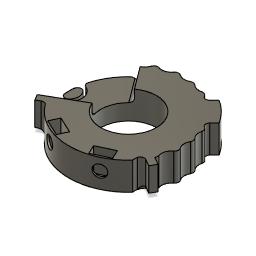
thumbwheelSmall (Autodesk Fusion 360 design; units mm, degrees)
Autodesk Fusion 360 part; units mm, degrees
sketch "Sketch1" plane through (0, 0, 0) normal (0, 1, 0) x (1, 0, 0)
  circle A0 centre (0, 0) radius 7
  circle A1 centre (0, 0) radius 15
  line L0 (0, -32.8401) -> (0, 23.247)
  line L1 (-28.2843, 0) -> (28.2843, 0)
  line L2 (6.3393, 13.5946) -> (-6.3393, -13.5946)
  line L3 (6.3393, 13.5946) -> (-6.3393, -13.5946)
  line L4 (-6.3393, 13.5946) -> (6.3393, -13.5946)
  circle A2 centre (-15, 0) radius 2.5
  circle A3 centre (-15, 0) radius 3.25
  circle A4 centre (0, 16.5) radius 2.5
  circle A5 centre (4.2705, 15.9378) radius 2.5
  circle A6 centre (8.25, 14.2894) radius 2.5
  circle A7 centre (11.6673, 11.6673) radius 2.5
  circle A8 centre (14.2894, 8.25) radius 2.5
  circle A9 centre (15.9378, 4.2705) radius 2.5
  circle A10 centre (16.5, 0) radius 2.5
  circle A11 centre (0, 0) radius 16.5
  circle A12 centre (-4.9423, 15.7424) radius 2.5
  circle A13 centre (15.7424, -4.9423) radius 2.5
  circle A14 centre (-9.4307, 13.5393) radius 2.5
  circle A15 centre (13.5393, -9.4307) radius 2.5
  line L5 (-4.0888, -14.0924) -> (-8.1672, -12.1906)
  line L6 (-8.1672, -12.1906) -> (-7.1106, -9.9248)
  line L7 (-7.1106, -9.9248) -> (-3.0322, -11.8266)
  line L8 (-3.0322, -11.8266) -> (-4.0888, -14.0924)
  line L9 (-4.0888, -14.0924) -> (-7.1106, -9.9248) construction
  line L10 (-8.1672, -12.1906) -> (-3.0322, -11.8266) construction
  line L11 (4.0888, -14.0924) -> (8.1672, -12.1906)
  line L12 (7.1106, -9.9248) -> (3.0322, -11.8266)
  line L13 (4.0888, -14.0924) -> (7.1106, -9.9248) construction
  line L14 (3.0322, -11.8266) -> (4.0888, -14.0924)
  line L15 (8.1672, -12.1906) -> (3.0322, -11.8266) construction
  line L16 (8.1672, -12.1906) -> (7.1106, -9.9248)
  line L17 (0, 0) -> (11.6673, 11.6673)
  line L18 (12.0629, 7.1131) -> (7.1131, 12.0629)
  line L19 (7.1131, 12.0629) -> (11.2717, 16.2214)
  line L20 (11.2717, 16.2214) -> (16.2214, 11.2717)
  line L21 (16.2214, 11.2717) -> (12.0629, 7.1131)
  line L22 (12.0629, 7.1131) -> (11.2717, 16.2214) construction
  line L23 (7.1131, 12.0629) -> (16.2214, 11.2717) construction
  point P0 (-5.5997, -12.0086)
  point P1 (6.3393, -13.5946)
  point P2 (6.3393, -13.5946)
  point P3 (5.5997, -12.0086)
  point P4 (11.6673, 11.6673)
  dimension "d1" = 14
  dimension "d2" = 30
  dimension "d3" = 25
  dimension "d6" = 5
  dimension "d7" = 6.5
  dimension "d8" = 5
  dimension "d10" = -90
  dimension "d36" = 5
  dimension "d37" = 5
  dimension "d38" = 5
  dimension "d39" = 5
  dimension "d47" = 4.5
  dimension "d48" = 2.5
  dimension "d49" = 0.5
  dimension "d60" = 45
  dimension "d61" = 33
  dimension "d62" = 7
  constraint coincident A0.centre A1.centre
  constraint concentric A0 A1
  constraint coincident A0.centre L0
  constraint coincident A0.centre L1
  constraint vertical L0
  constraint horizontal L1
  constraint coincident A0.centre L2
  constraint symmetric L0 L2.start L4.start
  constraint symmetric L0 L2.end P2
  constraint coincident A1 L4.start
  constraint coincident A1 L2.start
  constraint coincident A1 L2.end
  constraint coincident L1 A2.centre
  constraint coincident A1 A2.centre
  constraint concentric A2 A3
  constraint coincident L0 A4.centre
  constraint concentric A0 A11
  constraint coincident A10.centre A11
  constraint coincident A11 A12.centre
  constraint tangent A4 A12
  constraint coincident A11 A13.centre
  constraint coincident A11 A14.centre
  constraint tangent A12 A14
  constraint tangent A10 A13
  constraint coincident A11 A15.centre
  constraint tangent A13 A15
  constraint coincident L3 A0.centre
  constraint perpendicular L5 L6
  constraint parallel L5 L7
  constraint parallel L6 L8
  constraint coincident L9 P0
  constraint coincident L10 P0
  constraint coincident L2 P0
  constraint perpendicular L3 L7
  constraint symmetric L0 L5.start L11.start
  constraint symmetric L0 L5.end L11.end
  constraint symmetric L0 L6.end L12.start
  constraint symmetric L0 L7.end L12.end
  constraint symmetric L0 P0 P3
  constraint coincident P4 A7.centre
  constraint perpendicular L18 L19
  constraint parallel L18 L20
  constraint parallel L19 L21
  constraint coincident A8 L18.start
  constraint coincident L22 P4
  constraint coincident L23 P4
  constraint perpendicular L17 L20
  constraint coincident L3 P0
  measures "d1" diameter of A0
  measures "d2" diameter of A1
  measures "d3" angle of L0 L2
  measures "d6" diameter of A2
  measures "d7" diameter of A3
  measures "d8" diameter of A4
  measures "d36" diameter of A12
  measures "d37" diameter of A13
  measures "d38" diameter of A14
  measures "d39" diameter of A15
  measures "d47" distance of L6.end L7.end
  measures "d48" distance of L5.end L6.end
  measures "d49" distance of L2.end L5
  measures "d60" angle of L1 L17
  measures "d61" diameter of A11
  measures "d62" distance of L19.end L20.end
extrude "Extrude1" add sketch "Sketch1" along normal blind 7 contours A0 A1 L1 L4 A10 A13 A15 L11 L12 L16 | A0 A1 L1 A8 A9 A10 L17 L18 | A0 L2 L3 A6 L17 L18 | A0 A1 L0 L4 L11 L12 L14 | A0 A1 L0 L2 L3 A4 A5 A6 | A1 A6 A7 L17 L18 | A1 A7 A8 L17 L18 | A0 A1 L0 L2 L3 L5 L7 L8 | A0 A1 L0 L4 A4 A12 | A0 A1 L1 L4 A3 A14 | A0 A1 L1 L2 L3 A3 L5 L6 L7 | A1 A7 L17 | A1 A7 L17 | A1 A8 L21 | A1 A6 L19 | A1 A6 A7 A11 L17 | A1 A6 A7 | A1 A7 A8 | A1 A7 A8 A11 L17 | A1 A7 A8 A11 L21 | A1 A6 A7 A11 L19 | A1 L1 A2 | A1 L1 A2 | A6 A7 A11 | A7 A8 A11 picked at (12.3821, 7.9516) picked at (9.9243, 12.8711) picked at (12.8711, 9.9243) makes body 1 at (8.1025, 7, -7.9791) makes body 2 at (-12.801, 2.3333, -1.1893)
sketch "Sketch2" plane through (0, 0, 0) normal (0, -1, 0) x (1, 0, 0)
  arc A0 (8.9269, -13.8766) -> (13.8766, -8.9269) centre (0, 0) ccw
  line L0 (13.8766, -8.9269) -> (12.0629, -7.1131)
  arc A1 (13.8369, -5.7913) -> (12.0629, -7.1131) centre (14.2894, -8.25) ccw
  arc A2 (13.8369, -5.7913) -> (13.8793, -5.6891) centre (0, 0) ccw
  arc A3 (14.8644, -2.0127) -> (13.8793, -5.6891) centre (15.9378, -4.2705) ccw
  arc A4 (14.8644, -2.0127) -> (14.8788, -1.9031) centre (0, 0) ccw
  arc A5 (14.8788, 1.9031) -> (14.8788, -1.9031) centre (16.5, 0) ccw
  arc A6 (14.8788, 1.9031) -> (14.7657, 2.641) centre (0, 0) ccw
  arc A7 (13.6256, 6.2724) -> (14.7657, 2.641) centre (15.7424, 4.9423) ccw
  arc A8 (13.6256, 6.2724) -> (13.2967, 6.9425) centre (0, 0) ccw
  arc A9 (11.1212, 10.0657) -> (13.2967, 6.9425) centre (13.5393, 9.4307) ccw
  arc A10 (11.1212, 10.0657) -> (-14.6479, 3.2309) centre (0, 0) ccw
  arc A11 (-14.6479, -3.2309) -> (-14.6479, 3.2309) centre (-15, 0) ccw
  arc A12 (-14.6479, -3.2309) -> (-10.0657, -11.1212) centre (0, 0) ccw
  arc A13 (-6.9425, -13.2967) -> (-10.0657, -11.1212) centre (-9.4307, -13.5393) ccw
  arc A14 (-6.9425, -13.2967) -> (-6.2724, -13.6256) centre (0, 0) ccw
  arc A15 (-2.641, -14.7657) -> (-6.2724, -13.6256) centre (-4.9423, -15.7424) ccw
  arc A16 (-2.641, -14.7657) -> (-1.9031, -14.8788) centre (0, 0) ccw
  arc A17 (1.9031, -14.8788) -> (-1.9031, -14.8788) centre (0, -16.5) ccw
  arc A18 (1.9031, -14.8788) -> (2.0127, -14.8644) centre (0, 0) ccw
  arc A19 (5.6891, -13.8793) -> (2.0127, -14.8644) centre (4.2705, -15.9378) ccw
  arc A20 (5.6891, -13.8793) -> (5.7913, -13.8369) centre (0, 0) ccw
  arc A21 (7.1131, -12.0629) -> (5.7913, -13.8369) centre (8.25, -14.2894) ccw
  line L1 (7.1131, -12.0629) -> (8.9269, -13.8766)
  circle A22 centre (0, 0) radius 7
  line L2 (-8.1672, 12.1906) -> (-4.0888, 14.0924)
  line L3 (-4.0888, 14.0924) -> (-3.0322, 11.8266)
  line L4 (-3.0322, 11.8266) -> (-7.1106, 9.9248)
  line L5 (-7.1106, 9.9248) -> (-8.1672, 12.1906)
  line L6 (7.1106, 9.9248) -> (3.0322, 11.8266)
  line L7 (3.0322, 11.8266) -> (4.0888, 14.0924)
  line L8 (4.0888, 14.0924) -> (8.1672, 12.1906)
  line L9 (8.1672, 12.1906) -> (7.1106, 9.9248)
  arc A23 (-14.7917, -2.4913) -> (-14.7917, 2.4913) centre (-15, 0) ccw
  arc A24 (-14.7917, 2.4913) -> (-14.7917, -2.4913) centre (0, 0) ccw
  circle A25 centre (0, 0) radius 15
  constraint concentric A0 A25
extrude "Extrude2" add sketch "Sketch2" against normal blind 1 contours A11 A23 A25 | L2 L3 L4 L5 | L6 L7 L8 L9 bodies 1 2
sketch "Sketch3" plane through (0, 7, 0) normal (0, 1, 0) x (-1, 0, 0)
  arc A0 (-5.7913, -13.8369) -> (-5.6891, -13.8793) centre (0, 0) ccw
  arc A1 (-2.0127, -14.8644) -> (-5.6891, -13.8793) centre (-4.2705, -15.9378) ccw
  arc A2 (-2.0127, -14.8644) -> (-1.9031, -14.8788) centre (0, 0) ccw
  arc A3 (1.9031, -14.8788) -> (-1.9031, -14.8788) centre (0, -16.5) ccw
  arc A4 (14.6479, 3.2309) -> (14.6479, -3.2309) centre (15, 0) ccw
  arc A5 (10.0657, -11.1212) -> (14.6479, -3.2309) centre (0, 0) ccw
  circle A6 centre (0, 0) radius 12.5
  line L0 (0, 0) -> (14.6479, -3.2309)
  arc A7 (6.2724, -13.6256) -> (2.641, -14.7657) centre (4.9423, -15.7424) ccw
  arc A8 (10.0657, -11.1212) -> (6.9425, -13.2967) centre (9.4307, -13.5393) ccw
  line L1 (0, 0) -> (11.9795, 9.0272)
  line L2 (0, 0) -> (0, 15)
  line L3 (0, 0) -> (10.417, -14.0619)
  line L4 (7.1106, 9.9248) -> (3.0322, 11.8266)
  line L5 (4.0888, 14.0924) -> (8.1672, 12.1906)
  line L6 (8.1672, 12.1906) -> (7.1106, 9.9248)
  arc A9 (-5.7913, -13.8369) -> (-7.1131, -12.0629) centre (-8.25, -14.2894) ccw
  arc A10 (1.9031, -14.8788) -> (2.641, -14.7657) centre (0, 0) ccw
  arc A11 (-13.8766, -8.9269) -> (-8.9269, -13.8766) centre (0, 0) ccw
  line L7 (-8.9269, -13.8766) -> (-7.1131, -12.0629)
  arc A12 (6.2724, -13.6256) -> (6.9425, -13.2967) centre (0, 0) ccw
  arc A13 (-13.2967, 6.9425) -> (-11.1212, 10.0657) centre (-13.5393, 9.4307) ccw
  arc A14 (-13.2967, 6.9425) -> (-13.6256, 6.2724) centre (0, 0) ccw
  arc A15 (-14.7657, 2.641) -> (-13.6256, 6.2724) centre (-15.7424, 4.9423) ccw
  arc A16 (-14.7657, 2.641) -> (-14.8788, 1.9031) centre (0, 0) ccw
  arc A17 (-14.8788, -1.9031) -> (-14.8788, 1.9031) centre (-16.5, 0) ccw
  arc A18 (-14.8788, -1.9031) -> (-14.8644, -2.0127) centre (0, 0) ccw
  arc A19 (-13.8793, -5.6891) -> (-14.8644, -2.0127) centre (-15.9378, -4.2705) ccw
  arc A20 (-13.8793, -5.6891) -> (-13.8369, -5.7913) centre (0, 0) ccw
  arc A21 (-12.0629, -7.1131) -> (-13.8369, -5.7913) centre (-14.2894, -8.25) ccw
  line L8 (-12.0629, -7.1131) -> (-13.8766, -8.9269)
  circle A22 centre (0, 0) radius 7
  line L9 (3.0322, 11.8266) -> (4.0888, 14.0924)
  line L10 (-3.0322, 11.8266) -> (-7.1106, 9.9248)
  line L11 (-7.1106, 9.9248) -> (-8.1672, 12.1906)
  line L12 (-8.1672, 12.1906) -> (-4.0888, 14.0924)
  line L13 (-4.0888, 14.0924) -> (-3.0322, 11.8266)
  circle A23 centre (0, 0) radius 7
  arc A24 (14.6479, 3.2309) -> (-11.1212, 10.0657) centre (0, 0) ccw
  dimension "d46" = 53
  constraint coincident A4.end A5.end
  constraint coincident A0.centre A2.centre
  constraint coincident A5 L1.end
  constraint coincident A5 L2.end
  constraint vertical L2
  measures "d46" angle of L1 L2
extrude "Extrude3" cut sketch "Sketch3" 1 faces at (-14.1512, 7, 0) against normal blind 3 contours A4 A5 A6 L0 A8 L3 | A6 L0 L3 A22 A23 | A4 A6 L0 L1 A22 A23 | A4 A6 L0 | A4 A6 L1 A24 on bodies 1 bodies 1
fillet "Fillet1" radius 1 5 edges at (14.8788, 3.5, -1.9031) (14.8644, 3.5, -2.0127) (13.8793, 3.5, -5.6891) (13.8369, 3.5, -5.7913) (14.8788, 3.5, 1.9031) on bodies 1
fillet "Fillet1" radius 1 14 edges at (5.7913, 3.5, -13.8369) (5.6891, 3.5, -13.8793) (2.0127, 3.5, -14.8644) (1.9031, 3.5, -14.8788) (14.7657, 3.5, 2.641) (-10.0657, 2, -11.1212) (12.0629, 3.5, -7.1131) (7.1131, 3.5, -12.0629) (13.6256, 3.5, 6.2724) (13.2967, 3.5, 6.9425) (-1.9031, 3.5, -14.8788) (-2.641, 3.5, -14.7657) (-6.2724, 3.5, -13.6256) (-6.9425, 3.5, -13.2967) on bodies 1
sketch "Sketch4" plane through (0, 4, 0) normal (0, 1, 0) x (-1, 0, 0)
  arc A0 (10.4393, -10.7713) -> (14.6479, -3.2309) centre (0, 0) ccw
  line L0 (6.4435, 2.7351) -> (5.5904, 4.2127)
  line L1 (5.5904, 4.2127) -> (14.345, 9.2672)
  line L2 (14.345, 9.2672) -> (15.1981, 7.7896)
  line L3 (15.1981, 7.7896) -> (6.4435, 2.7351)
  line L4 (0, -19) -> (0, 26)
  line L5 (-15.1981, 7.7896) -> (-6.4435, 2.7351)
  line L6 (-14.345, 9.2672) -> (-15.1981, 7.7896)
  line L7 (-5.5904, 4.2127) -> (-14.345, 9.2672)
  line L8 (-6.4435, 2.7351) -> (-5.5904, 4.2127)
  line L9 (14.7716, 8.5284) -> (0, 0)
  line L10 (0, 0) -> (-14.7716, 8.5284)
  line L11 (11.9795, 9.0272) -> (5.5904, 4.2127)
  arc A1 (14.6479, 3.2309) -> (14.6479, -3.2309) centre (15, 0) ccw
  arc A2 (9.654, -11.0493) -> (10.4393, -10.7713) centre (9.7433, -10.0533) ccw
  arc A3 (14.6479, 3.2309) -> (11.9795, 9.0272) centre (0, 0) ccw
  arc A4 (4.1668, -5.6248) -> (5.5904, 4.2127) centre (0, 0) ccw
  line L12 (4.1668, -5.6248) -> (8.3572, -11.2815)
  arc A5 (9.654, -11.0493) -> (8.3572, -11.2815) centre (9.4307, -13.5393) ccw
  point P0 (-17.1982, 3.236)
  dimension "d44" = 60
  constraint perpendicular L0 L1
  constraint parallel L0 L2
  constraint parallel L1 L3
  constraint vertical L4
  constraint symmetric L0.start L4 L5.end
  constraint symmetric L0.end L4 L7.start
  constraint symmetric L1.end L4 L6.start
  constraint symmetric L2.end L4 L5.start
  constraint coincident A0.centre L4
  constraint coincident A0.centre L9.end
  constraint midpoint L6 L10.end
  constraint midpoint L2 L9.start
  constraint perpendicular L0 L9
  constraint coincident L0.start A4
  constraint coincident L0.end L1.start
  measures "d44" angle of L4 L9
extrude "Extrude4" add sketch "Sketch4" along normal blind 3 contours L2 L3 L9 A3 | L3 L9 A3 A4 | L1 L2 L9 A3 | L1 L9 A3 A4 | L1 L11 A3 | L5 L6 L8 L10 | L6 L7 L8 L10 bodies 1
extrude "Extrude5" add 2 faces at (-14.1296, 4, 8.2673) (14.1773, 4, 8.0004) along direction (0, -1, 0) blind 3 on bodies 1 bodies 1
fillet "Fillet3" radius 2 1 edges at (-12.9904, 1, 7.5) on bodies 1
fillet "Fillet6" radius 1 8 edges at (11.6984, 4, 7.7392) (-12.5428, 3.5, 8.2267) (-9.9197, 4, 4.7421) (-6.262, 4, -8.4531) (-14.7917, 2.5, -2.4913) (-14.6479, 2.5, -3.2309) (-14.6479, 2.5, 3.2309) (-14.7917, 2.5, 2.4913) on bodies 1
sketch "Sketch6" plane through (0, 0, 0) normal (0, -1, 0) x (1, 0, 0)
  arc A0 (11.1212, 10.0657) -> (-12.0343, 8.954) centre (0, 0) ccw
  arc A1 (-12.0343, 8.954) -> (-13.3959, 6.7491) centre (0, 0) ccw
  arc A2 (11.1212, 10.0657) -> (12.7555, 7.0568) centre (13.5393, 9.4307) ccw
  arc A3 (-13.3959, 6.7491) -> (-10.4393, -10.7713) centre (0, 0) ccw
  arc A4 (-10.4393, -10.7713) -> (-9.654, -11.0493) centre (-9.7433, -10.0533) ccw
  arc A5 (-7.0568, -12.7555) -> (-9.654, -11.0493) centre (-9.4307, -13.5393) ccw
  arc A6 (-2.9121, -14.2836) -> (-5.7743, -13.385) centre (-4.9423, -15.7424) ccw
  arc A7 (1.268, -14.3454) -> (-1.5, -14.5) centre (0, -16.5) ccw
  arc A8 (1.268, -14.3454) -> (2.4881, -14.1848) centre (1.7751, -13.4836) ccw
  arc A9 (4.9376, -13.5284) -> (2.4881, -14.1848) centre (4.2705, -15.9378) ccw
  arc A10 (4.9376, -13.5284) -> (6.0746, -13.0575) centre (5.2045, -12.5647) ccw
  arc A11 (6.2326, -12.8129) -> (6.0746, -13.0575) centre (8.25, -14.2894) ccw
  arc A12 (7.7467, -12.6964) -> (6.2326, -12.8129) centre (7.0396, -13.4035) ccw
  line L0 (7.7467, -12.6964) -> (8.9269, -13.8766)
  arc A13 (8.9269, -13.8766) -> (13.8766, -8.9269) centre (0, 0) ccw
  line L1 (13.8766, -8.9269) -> (12.6964, -7.7467)
  arc A14 (12.8129, -6.2326) -> (12.6964, -7.7467) centre (13.4035, -7.0396) ccw
  arc A15 (13.0575, -6.0746) -> (12.8129, -6.2326) centre (14.2894, -8.25) ccw
  arc A16 (13.0575, -6.0746) -> (13.5284, -4.9376) centre (12.5647, -5.2045) ccw
  arc A17 (14.1848, -2.4881) -> (13.5284, -4.9376) centre (15.9378, -4.2705) ccw
  arc A18 (14.1848, -2.4881) -> (14.3454, -1.268) centre (13.4836, -1.7751) ccw
  arc A19 (14.5, 1.5) -> (14.3454, -1.268) centre (16.5, 0) ccw
  arc A20 (14.5, 1.5) -> (14.2836, 2.9121) centre (13.7, 2.1) ccw
  arc A21 (13.385, 5.7743) -> (14.2836, 2.9121) centre (15.7424, 4.9423) ccw
  arc A22 (13.385, 5.7743) -> (12.7555, 7.0568) centre (12.442, 6.1072) ccw
  circle A23 centre (0, 0) radius 7
  arc A24 (-7.0568, -12.7555) -> (-5.7743, -13.385) centre (-6.1072, -12.442) ccw
  arc A25 (-2.9121, -14.2836) -> (-1.5, -14.5) centre (-2.1, -13.7) ccw
sketch "Sketch7" plane through (-5.0714, 0, 10.8757) normal (-0.422618, 0, 0.906308) x (0.906308, 0, 0.422618)
  line L0 (2.25, 1) -> (2.25, 7)
  line L1 (2.25, 7) -> (-2.25, 7)
  circle A0 centre (0, 4) radius 1.5
  line L2 (-2.25, 7) -> (-2.25, 1)
  line L3 (-2.25, 1) -> (2.25, 1)
  point P0 (0, 7)
  point P1 (2.25, 4)
  dimension "d52" = 3
  constraint midpoint L1 P0
  constraint midpoint L0 P1
  constraint vertical A0.centre P0
  constraint horizontal A0.centre P1
  measures "d52" diameter of A0
extrude "Extrude8" cut sketch "Sketch7" along normal blind 5 contours A0 bodies 1
sketch "Sketch8" plane through (5.0714, 0, 10.8757) normal (0.422618, 0, 0.906308) x (0.906308, 0, -0.422618)
  line L0 (2.25, 1) -> (2.25, 7)
  line L1 (2.25, 7) -> (-2.25, 7)
  line L2 (-2.25, 7) -> (-2.25, 1)
  circle A0 centre (0, 4) radius 1.5
  line L3 (-2.25, 1) -> (2.25, 1)
  point P0 (0, 7)
  point P1 (2.25, 4)
  dimension "d55" = 3
  constraint midpoint L1 P0
  constraint midpoint L0 P1
  constraint horizontal A0.centre P1
  constraint vertical A0.centre P0
  measures "d55" diameter of A0
extrude "Extrude9" cut sketch "Sketch8" along normal blind 5 contours A0 bodies 1
fillet "Fillet9" radius 1 2 edges at (13.042, 1, 6.9071) (11.6822, 1, 7.757) on bodies 1
